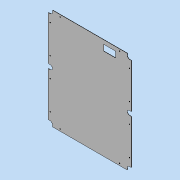
# Autodesk Inventor part: Bottom_Plate
Saved by Autodesk Inventor 2020 (Build 240168000, 168)
## iProperties
Created: 2021-06-14
Part Number: Bottom_Plate
Material: 一般
Document SubType Name: Sheet Metal
Designer: magnarecta
Density: 1 g/cm^3
Sheet Metal Rule: Default_mm
Appearance: 既定
Author: magnarecta
Autodesk Inventor part; units mm, degrees
ref_plane "YZ Plane" through (0, 0, 0) normal (1, 0, 0) x (0, 1, 0)
ref_plane "XZ Plane" through (0, 0, 0) normal (0, 1, 0) x (-1, 0, 0)
ref_plane "XY Plane" through (0, 0, 0) normal (0, 0, 1) x (1, 0, 0)
sketch "スケッチ1" plane through (0, 0, 0) normal (0, 0, 1) x (1, 0, 0)
  line L0 (210, -255) -> (-210, -255)
  line L1 (-210, -255) -> (-210, 255)
  line L2 (-210, 255) -> (210, 255)
  line L3 (210, 255) -> (210, -255)
  line L4 (210, -255) -> (-210, 255) construction
  line L5 (-210, -255) -> (210, 255) construction
  point P0 (0, 0)
  dimension "d0" = 510
  dimension "d1" = 420
  measures "d0" distance of L0.end L1.end
  measures "d1" distance of L0.start L0.end
extrude "プレート1" add sketch "スケッチ1" along normal blind 1.2
sketch "スケッチ2" plane through (0, 0, 1.2) normal (0, 0, 1) x (1, 0, 0)
  line L0 (-210, -255) -> (-210, 255) projected
  line L1 (210, -255) -> (-210, -255) projected
  line L2 (210, 255) -> (210, -255) projected
  line L3 (-210, 255) -> (210, 255) projected
  line L4 (189, 234) -> (189, -234)
  line L5 (189, -234) -> (-189, -234)
  line L6 (-189, -234) -> (-189, 234)
  line L7 (-189, 234) -> (189, 234)
  line L8 (200, 245) -> (200, -245)
  line L9 (200, -245) -> (-200, -245)
  line L10 (-200, -245) -> (-200, 245)
  line L11 (-200, 245) -> (200, 245)
  circle A0 centre (-200, 245) radius 11
  circle A1 centre (-200, -245) radius 11
  circle A2 centre (200, -245) radius 11
  circle A3 centre (200, 245) radius 11
  circle A4 centre (-200, 0) radius 11
  circle A5 centre (200, 0) radius 11
  line L12 (-296, 11) -> (393, 11)
  line L13 (393, 11) -> (393, -11)
  line L14 (393, -11) -> (-296, -11)
  line L15 (-296, -11) -> (-296, 11)
  line L16 (-292, 336) -> (-189, 336)
  line L17 (-189, 336) -> (-189, -344)
  line L18 (-189, -344) -> (-292, -344)
  line L19 (-292, -344) -> (-292, 336)
  line L20 (354, -311) -> (189, -311)
  line L21 (189, -311) -> (189, 377)
  line L22 (189, 377) -> (354, 377)
  line L23 (354, 377) -> (354, -311)
  line L24 (-371, 292) -> (290, 292)
  line L25 (290, 292) -> (290, 234)
  line L26 (290, 234) -> (-371, 234)
  line L27 (-371, 234) -> (-371, 292)
  line L28 (-371, -325) -> (335, -325)
  line L29 (335, -325) -> (335, -234)
  line L30 (335, -234) -> (-371, -234)
  line L31 (-371, -234) -> (-371, -325)
  point P0 (0, 0)
  point P1 (200, 11)
  point P2 (200, -11)
  point P3 (210, -11)
  point P4 (210, 11)
  point P5 (210, -234)
  point P6 (200, -234)
  point P7 (189, -245)
  point P8 (189, -255)
  point P9 (-189, -245)
  point P10 (-200, -234)
  point P11 (-210, -234)
  point P12 (-189, -255)
  point P13 (-200, 11)
  point P14 (-210, 11)
  point P15 (-210, -11)
  point P16 (-200, -11)
  point P17 (-210, 234)
  point P18 (-200, 234)
  point P19 (-189, 245)
  point P20 (-189, 255)
  point P21 (189, 245)
  point P22 (200, 234)
  point P23 (210, 234)
  point P24 (189, 255)
  point P25 (210, 249.5826)
  point P26 (195.4174, 255)
  point P27 (-189, 245)
  point P28 (189, 245)
  point P29 (200, 234)
  point P30 (200, 234)
  point P31 (204.5826, 255)
  dimension "d3" = 21
  dimension "d4" = 10
  dimension "d5" = 22
  dimension "d6" = 22
  dimension "d7" = 22
  dimension "d8" = 22
  dimension "d9" = 22
  dimension "d10" = 22
  constraints: 56 end point, 10 parallel, 6 centre point, 6 tangent, 5 horizontal, 5 perpendicular, 4 coincident, 2 midpoint, 1 point on line, 6 other
  measures "d3" distance between parallel lines of L3 L7
  measures "d4" distance between parallel lines of L3 L11
  measures "d5" diameter of A0
  measures "d6" diameter of A1
  measures "d7" diameter of A2
  measures "d8" diameter of A3
  measures "d9" diameter of A4
  measures "d10" diameter of A5
extrude "押し出し1" cut sketch "スケッチ2" against normal blind 10 contours L0 A1 L1 | L0 A1 L10 L9 L1 | L0 L30 A1 | A1 L17 L1 | A1 L9 L10 | L0 A4 L14 | A4 L0 L10 | L10 A4 | L21 A2 L1 | A2 L8 L9 | L9 L8 A2 L2 L1 | A4 L0 L12 | L30 L2 A2 | A0 L0 L3 L11 L10 | L26 L0 A0 | L10 L11 A0 | A2 L2 L1 | A5 L8 | L8 A5 L2 | A5 L2 L14 | L26 L27 L24 L19 | L19 L24 L17 L3 A0 L0 L26 | A0 L0 | A0 L3 L17 | L12 L2 A5 | L0 L3 A0 | A3 L3 L2 L8 L11 | L21 L3 A3 | L11 L8 A3 | L3 A0 | L17 L24 L21 L3 | A3 L2 L26 | A3 L3 | L3 L21 L24 L25 L26 L2 A3 | L2 A3 | L3 L2 A3
fillet "フィレット1" radius 2 12 edges at (-210, 11, 0.6) (-210, -11, 0.6) (-210, 234, 0.6) (-189, 255, 0.6) (189, 255, 0.6) (210, 234, 0.6) (210, 11, 0.6) (210, -11, 0.6) (210, -234, 0.6) (189, -255, 0.6) (-210, -234, 0.6) (-189, -255, 0.6)
sketch "スケッチ3" plane through (0, 0, 1.2) normal (0, 0, 1) x (1, 0, 0)
  arc A0 (-189, -253) -> (-187, -255) centre (-187, -253) ccw projected
  line L0 (187, -255) -> (-187, -255) projected
  arc A1 (187, -255) -> (189, -253) centre (187, -253) ccw projected
  line L1 (189, -253) -> (189, -245) projected
  arc A2 (200, -234) -> (189, -245) centre (200, -245) ccw projected
  line L2 (200, -234) -> (208, -234) projected
  arc A3 (208, -234) -> (210, -232) centre (208, -232) ccw projected
  line L3 (210, -13) -> (210, -232) projected
  arc A4 (210, -13) -> (208, -11) centre (208, -13) ccw projected
  line L4 (208, -11) -> (200, -11) projected
  arc A5 (200, 11) -> (200, -11) centre (200, 0) ccw projected
  line L5 (200, 11) -> (208, 11) projected
  arc A6 (208, 11) -> (210, 13) centre (208, 13) ccw projected
  line L6 (210, 232) -> (210, 13) projected
  arc A7 (210, 232) -> (208, 234) centre (208, 232) ccw projected
  line L7 (208, 234) -> (200, 234) projected
  arc A8 (189, 245) -> (200, 234) centre (200, 245) ccw projected
  line L8 (189, 245) -> (189, 253) projected
  arc A9 (189, 253) -> (187, 255) centre (187, 253) ccw projected
  line L9 (-187, 255) -> (187, 255) projected
  arc A10 (-187, 255) -> (-189, 253) centre (-187, 253) ccw projected
  line L10 (-189, 253) -> (-189, 245) projected
  arc A11 (-200, 234) -> (-189, 245) centre (-200, 245) ccw projected
  line L11 (-200, 234) -> (-208, 234) projected
  arc A12 (-208, 234) -> (-210, 232) centre (-208, 232) ccw projected
  line L12 (-210, 13) -> (-210, 232) projected
  arc A13 (-210, 13) -> (-208, 11) centre (-208, 13) ccw projected
  line L13 (-208, 11) -> (-200, 11) projected
  arc A14 (-200, -11) -> (-200, 11) centre (-200, 0) ccw projected
  line L14 (-200, -11) -> (-208, -11) projected
  arc A15 (-208, -11) -> (-210, -13) centre (-208, -13) ccw projected
  line L15 (-210, -232) -> (-210, -13) projected
  arc A16 (-210, -232) -> (-208, -234) centre (-208, -232) ccw projected
  line L16 (-208, -234) -> (-200, -234) projected
  arc A17 (-189, -245) -> (-200, -234) centre (-200, -245) ccw projected
  line L17 (-189, -245) -> (-189, -253) projected
  line L18 (200, -245) -> (-200, -245)
  line L19 (-200, -245) -> (-200, 245)
  line L20 (-200, 245) -> (200, 245)
  line L21 (200, 245) -> (200, -245)
  line L22 (200, -245) -> (-200, 245) construction
  line L23 (-200, -245) -> (200, 245) construction
  point P0 (0, 0)
  point P1 (-150, 245)
  point P2 (150, 245)
  point P3 (-200, 195)
  point P4 (-200, 50)
  point P5 (200, 50)
  point P6 (200, 195)
  point P7 (200, -195)
  point P8 (200, -50)
  point P9 (150, -245)
  point P10 (-150, -245)
  point P11 (-200, -195)
  point P12 (-200, -50)
  dimension "d14" = 10
  dimension "d15" = 10
  dimension "d16" = 150
  dimension "d17" = 300
  dimension "d18" = 145
  dimension "d19" = 50
  dimension "d20" = 145
  dimension "d21" = 50
  constraints: 12 end point, 12 point on line, 4 horizontal alignment, 2 midpoint, 2 parallel, 2 vertical alignment, 1 horizontal, 1 perpendicular
  measures "d14" distance between parallel lines of L19 L12
  measures "d15" distance between parallel lines of L9 L20
  measures "d16" horizontal distance of point (-150, 245) point (0, 0)
  measures "d17" distance of point (150, 245) point (-150, 245)
  measures "d18" distance of point (-200, -50) point (-200, -195)
  measures "d19" distance from line of point (-200, -195) L18
  measures "d20" distance of point (-200, 195) point (-200, 50)
  measures "d21" distance from line of point (-200, 195) L20
hole "穴1" at (-150, 245, 1.2) at (150, 245, 1.2) at (-200, 195, 1.2) at (-200, 50, 1.2) at (200, 50, 1.2) at (200, 195, 1.2) at (200, -195, 1.2) at (200, -50, 1.2) at (150, -245, 1.2) at (-150, -245, 1.2) at (-200, -195, 1.2) at (-200, -50, 1.2) direction (0, 0, -1) diameter 4.5 depth 1.2 tip angle 118
sketch "スケッチ4" plane through (0, 0, 1.2) normal (0, 0, 1) x (1, 0, 0)
  line L0 (190, -235) -> (-190, -235)
  line L1 (-190, -235) -> (-190, 235)
  line L2 (-190, 235) -> (190, 235)
  line L3 (190, 235) -> (190, -235)
  line L4 (190, -235) -> (-190, 235) construction
  line L5 (-190, -235) -> (190, 235) construction
  line L6 (-187, 255) -> (187, 255) projected
  line L7 (-210, 13) -> (-210, 232) projected
  line L8 (70, 235) -> (130, 235)
  line L9 (130, 235) -> (130, 205)
  line L10 (130, 205) -> (70, 205)
  line L11 (70, 205) -> (70, 235)
  point P0 (0, 0)
  point P1 (100, 205)
  dimension "d29" = 20
  dimension "d30" = 20
  dimension "d31" = 30
  dimension "d32" = 60
  dimension "d33" = 100
  constraints: 20 end point, 4 parallel, 3 midpoint, 2 horizontal, 2 perpendicular, 1 point on line
  measures "d29" distance between parallel lines of L6 L2
  measures "d30" distance between parallel lines of L1 L7
  measures "d31" distance of L8.end L9.end
  measures "d32" distance of L9.end L10.end
  measures "d33" horizontal distance of point (100, 205) point (0, 0)
extrude "押し出し2" cut sketch "スケッチ4" against normal blind 10 contours L9 L10 L11 L2
equation "\"d27\" = Thickness"
equation "\"d2\" = Thickness"
equation "\"BendRadius\" = Thickness"
equation "\"BendReliefWidth\" = Thickness"
equation "\"BendReliefDepth\" = 0.5 * Thickness"
equation "\"CornerReliefSize\" = 4 * Thickness"
equation "\"MinimumRemnant\" = 2 * Thickness"
equation "\"TransitionRadius\" = BendRadius"
equation "\"JacobiRadiusSize\" = BendRadius"
equation "\"GapSize\" = Thickness"
equation "\"Thickness\" = 1.2"
